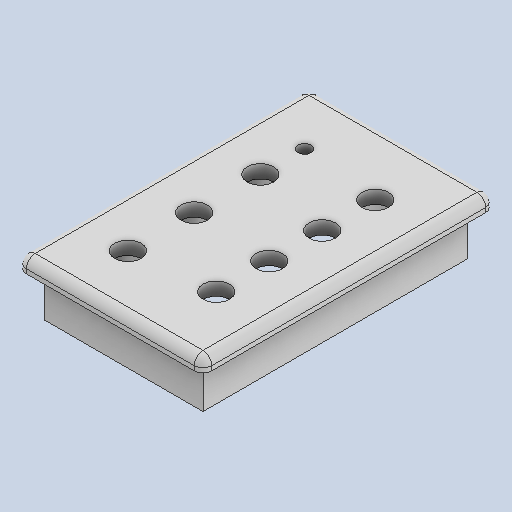
# Autodesk Inventor part: vstup
Saved by Autodesk Inventor 2025 (Build 290162000, 162)
## iProperties
Created: 2025-09-15
Part Number: vstup
Material: Generic
Document SubType Name: Modeling
Designer: Pravoslav
Density: 1 g/cm^3
Appearance: Default
Author: Pravoslav
Autodesk Inventor part; units mm, degrees
ref_plane "YZ Plane" through (0, 0, 0) normal (1, 0, 0) x (0, 1, 0)
ref_plane "XZ Plane" through (0, 0, 0) normal (0, 1, 0) x (-1, 0, 0)
ref_plane "XY Plane" through (0, 0, 0) normal (0, 0, 1) x (1, 0, 0)
sketch "Sketch1" plane through (0, 0, 0) normal (0, 1, 0) x (-1, 0, 0)
  line L0 (18, 30) -> (-18, 30)
  line L1 (-18, 30) -> (-18, -30)
  line L2 (-18, -30) -> (18, -30)
  line L3 (18, -30) -> (18, 30)
  line L4 (18, 30) -> (-18, -30) construction
  line L5 (-18, 30) -> (18, -30) construction
  circle A0 centre (9, 20) radius 3
  circle A1 centre (9, 5) radius 3
  circle A2 centre (-9, 18) radius 3
  circle A3 centre (-9, 6) radius 3
  circle A4 centre (-9, -6) radius 3
  circle A5 centre (-9, -18) radius 3
  circle A6 centre (9, -10) radius 3
  circle A7 centre (9, -20) radius 1.5
  line L6 (21, 33) -> (-21, 33)
  line L7 (-21, 33) -> (-21, -33)
  line L8 (-21, -33) -> (21, -33)
  line L9 (21, -33) -> (21, 33)
  line L10 (21, 33) -> (-21, -33) construction
  line L11 (-21, 33) -> (21, -33) construction
  point P0 (0, 0)
  dimension "d0" = 36
  dimension "d1" = 60
  dimension "d2" = 6
  dimension "d3" = 6
  dimension "d4" = 6
  dimension "d5" = 6
  dimension "d6" = 6
  dimension "d7" = 6
  dimension "d8" = 6
  dimension "d9" = 3
  dimension "d10" = 10
  dimension "d11" = 5
  dimension "d12" = 9
  dimension "d13" = 9
  dimension "d14" = 9
  dimension "d15" = 9
  dimension "d16" = 10
  dimension "d17" = 10
  dimension "d18" = 9
  dimension "d19" = 9
  dimension "d20" = 9
  dimension "d21" = 9
  dimension "d22" = 12
  dimension "d23" = 12
  dimension "d24" = 12
  dimension "d25" = 12
  dimension "d26" = 3
  dimension "d27" = 3
  constraints: 24 end point, 8 centre point, 4 midpoint, 4 parallel, 2 horizontal, 2 perpendicular
  measures "d0" distance of L2.end L1.end
  measures "d1" distance of L1.end L0.end
  measures "d2" diameter of A0
  measures "d3" diameter of A1
  measures "d4" diameter of A2
  measures "d5" diameter of A3
  measures "d6" diameter of A4
  measures "d7" diameter of A5
  measures "d8" diameter of A6
  measures "d9" diameter of A7
  measures "d10" distance from line of L0 A0.centre
  measures "d11" vertical distance of point (0, 0) A1.centre
  measures "d12" distance from line of L3 A0.centre
  measures "d13" distance from line of L3 A1.centre
  measures "d14" distance from line of L3 A7.centre
  measures "d15" distance from line of L3 A6.centre
  measures "d16" vertical distance of point (0, 0) A6.centre
  measures "d17" distance from line of L2 A7.centre
  measures "d18" distance from line of L1 A4.centre
  measures "d19" distance from line of L1 A5.centre
  measures "d20" distance from line of L1 A3.centre
  measures "d21" distance from line of L1 A2.centre
  measures "d22" distance from line of L0 A2.centre
  measures "d23" distance of A2.centre A3.centre
  measures "d24" distance of A4.centre A3.centre
  measures "d25" distance of A5.centre A4.centre
  measures "d26" distance between parallel lines of L9 L3
  measures "d27" distance between parallel lines of L2 L8
extrude "Extrusion1" add sketch "Sketch1" along normal blind 3 contours L3 L2 L1 L0 | L9 L8 L7 L6
sketch "Sketch2" plane through (0, 0, 0) normal (0, -1, 0) x (1, 0, 0)
  line L0 (18, 30) -> (-18, 30)
  line L1 (-18, 30) -> (-18, -30)
  line L2 (-18, -30) -> (18, -30)
  line L3 (18, -30) -> (18, 30)
  line L4 (18, 30) -> (-18, -30) construction
  line L5 (-18, 30) -> (18, -30) construction
  line L6 (16, 28) -> (-16, 28)
  line L7 (-16, 28) -> (-16, -28)
  line L8 (-16, -28) -> (16, -28)
  line L9 (16, -28) -> (16, 28)
  line L10 (16, 28) -> (-16, -28) construction
  line L11 (-16, 28) -> (16, -28) construction
  point P0 (0, 0)
  dimension "d30" = 36
  dimension "d31" = 60
  dimension "d32" = 2
  dimension "d33" = 2
  constraints: 24 end point, 4 midpoint, 4 parallel, 2 horizontal, 2 perpendicular
  measures "d30" distance of L2.end L1.end
  measures "d31" distance between parallel lines of L2 L0
  measures "d32" distance between parallel lines of L3 L9
  measures "d33" distance between parallel lines of L2 L8
extrude "Extrusion2" add sketch "Sketch2" along normal blind 10
fillet "Fillet1" radius 2 8 edges at (21, 3, 0) (0, 3, -33) (0, 3, 33) (-21, 3, 0) (21, 1.5, 33) (21, 1.5, -33) (-21, 1.5, -33) (-21, 1.5, 33)
body "Solid1"
